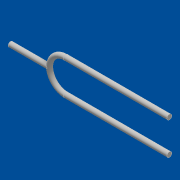
# Autodesk Inventor part: Y_ancla
Saved by Autodesk Inventor 2016 (Build 200138000, 138)
## iProperties
Created: 2017-05-13
Part Number: Y_ancla
Material: Generic
Document SubType Name: Modeling
Designer: Gian
Density: 1 g/cm^3
Appearance: Default
Author: Gian
Autodesk Inventor part; units mm, degrees
ref_plane "XZ Plane" through (0, 0, 0) normal (0, 1, 0) x (-1, 0, 0)
ref_plane "XY Plane" through (0, 0, 0) normal (0, 0, 1) x (1, 0, 0)
sketch "Sketch4" plane through (0, 0, 0) normal (1, 0, 0) x (0, 1, 0)
  circle A0 centre (20.1532, 0.0226) radius 9.525
  circle A1 centre (20.1532, 0.0226) radius 9.525
  dimension "d10" = 19.05
  dimension "d21" = 19.05
  constraints: 2 centre point, 1 coincident
  measures "d10" diameter of A0
  measures "d21" diameter of A1
sketch "Sketch5" plane through (0, 0, 0) normal (0, 1, 0) x (-1, 0, 0)
  line L0 (0, 9.5476) -> (0, -9.5024) projected
  line L1 (398.5, 0.0226) -> (0, 0.0226)
  arc A0 (398.5, 0.0226) -> (398.5, 125.0226) centre (398.5, 62.5226) ccw
  line L2 (398.5, 62.5226) -> (398.5, 125.0226) construction
  line L3 (398.5, 62.5226) -> (398.5, 0.0226) construction
  line L4 (398.5, 125.0226) -> (0, 125.0226)
  line L5 (461, 62.5226) -> (611, 62.5226)
  dimension "d14" = 398.5
  dimension "d15" = 125
  dimension "d18" = 150
  constraints: 10 end point, 3 horizontal, 3 point on circle, 1 centre point, 1 midpoint, 1 parallel, 1 point on line, 1 vertical
  measures "d14" distance of L1.start L1.end
  measures "d15" diameter of A0
  measures "d18" distance of L5.start L5.end
sweep "Sweep4" add profiles "Sketch4" path "Sketch5" path curves L1 A0 L4
ref_plane "Work Plane1" through (-461.6, 0, 0) normal (1, 0, 0) x (0, 1, 0)
sketch "Sketch8" plane through (-461.6, 0, 0) normal (1, 0, 0) x (0, 1, 0)
  circle A0 centre (20.1532, 125.0226) radius 9.525 projected
  circle A1 centre (20.1532, 0.0226) radius 9.525 projected
  line L0 (20.1532, 125.0226) -> (20.1532, 0.0226)
  circle A2 centre (20.1532, 62.5226) radius 9.525
  dimension "d24" = 19.05
  constraints: 2 end point, 1 centre point, 1 midpoint, 1 vertical
  measures "d24" diameter of A2
sweep "Sweep5" add profiles "Sketch8" path "Sketch5" path curves L5 contours A2 L0 | L0 A2
body "Solid4"
